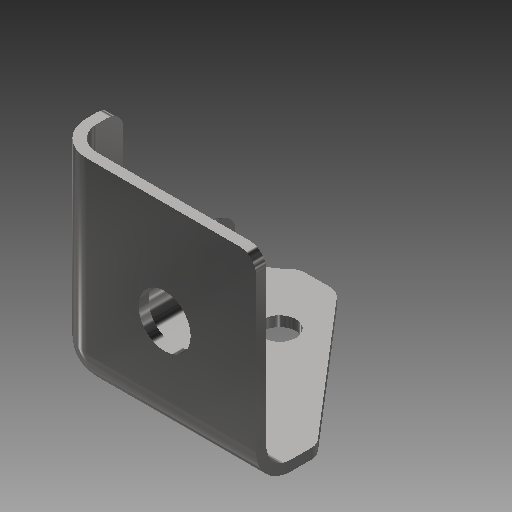
# Autodesk Inventor part: 314-06
Saved by Autodesk Inventor 2019 (Build 230136000, 136)
## iProperties
Company: Autodesk Inc.
Created: 2007-10-25
Part Number: 314-06
Document SubType Name: Modeling
Designer: Autodesk Inc.
Density: 7.85 g/cm^3
Mass: 90.2439 g
Surface Area: 99.9897 cm^2
Volume: 11.496 cm^3
Material: Steel
Description: CORNER BRACKET - L
Appearance: Steel - Polished
Component Category: Lower Component
Author: Inventor
Autodesk Inventor part; units mm, degrees
ref_plane "YZ Plane" through (0, 0, 0) normal (1, 0, 0) x (0, 1, 0)
ref_plane "XZ Plane" through (0, 0, 0) normal (0, 1, 0) x (-1, 0, 0)
ref_plane "XY Plane" through (0, 0, 0) normal (0, 0, 1) x (1, 0, 0)
sketch "Sketch1" plane through (0, 0, 0) normal (0, 0, 1) x (1, 0, 0)
  line L0 (-25, 25) -> (25, 25)
  line L1 (25, 25) -> (25, -25)
  line L2 (25, -25) -> (-25, -25)
  line L3 (-25, -25) -> (-25, 25)
  point P0 (0, 0)
  dimension "d0" = 50
  dimension "d1" = 50
  dimension "d2" = 25
  dimension "d3" = 25
  constraints: 8 end point, 2 parallel, 1 horizontal, 1 perpendicular
  measures "d0" distance of L2.end L0.start
  measures "d1" distance of L0.start L0.end
  measures "d2" distance from line of point (0, 0) L3
  measures "d3" distance from line of point (0, 0) L0
extrude "Extrusion1" add sketch "Sketch1" against normal blind 50
fillet "Fillet1" radius 8.5 3 edges at (0, -25, 0) (-25, 0, 0) (-25, -25, -25)
shell "Shell1" thickness 2.5 removed faces 3 at (-8.3333, 11.1667, -50) at (-8.3333, 25, -36.1667) at (25, 11.1667, -16.6667)
sketch "Sketch2" plane through (-25, -16.5, -8.5) normal (-1, 0, 0) x (0, 0, 1)
  line L0 (0, 41.5) -> (-41.5, 41.5) projected
  line L1 (-41.5, 41.5) -> (-41.5, 0) projected
  line L2 (-41.5, 6.5) -> (-6.5, 6.5)
  line L3 (-6.5, 6.5) -> (-6.5, 41.5)
  line L4 (-6.5, 41.5) -> (-41.5, 41.5)
  line L5 (-41.5, 41.5) -> (-41.5, 6.5)
  point P0 (8.5, 16.5)
  dimension "d8" = 35
  dimension "d9" = 35
  constraints: 8 end point, 2 parallel, 2 point on line, 1 horizontal, 1 perpendicular
  measures "d8" distance of L2.start L2.end
  measures "d9" distance from line of L2 L0.start
extrude "Extrusion2" cut sketch "Sketch2" against normal through all
sketch "Sketch3" plane through (-16.5, 25, 0) normal (0, 1, 0) x (1, 0, 0)
  line L0 (41.5, 0) -> (41.5, 2.5) projected
  line L1 (41.5, 15) -> (11.5, 50)
  line L2 (0, 50) -> (41.5, 50) projected
  line L3 (41.5, 50) -> (11.5, 50)
  line L4 (41.5, 50) -> (41.5, 15)
  point P0 (41.5, 33)
  point P1 (41.5, 8.5)
  point P2 (16.5, 0)
  point P3 (33, 50)
  point P4 (39, 50)
  dimension "d36" = 30
  dimension "d37" = 35
  constraints: 7 end point, 2 collinear, 2 point on line
  measures "d36" distance of L2.end L1.end
  measures "d37" distance of L2.end L1.start
extrude "Extrusion3" cut sketch "Sketch3" against normal through all
sketch "Sketch4" plane through (0, 0, 0) normal (0, 0, 1) x (1, 0, 0)
  line L0 (-5, -25) -> (25, -25) projected
  line L1 (-16.5, -25) -> (25, -25) projected
  line L2 (-16.5, -25) -> (-5, -25) projected
  line L3 (-25, 25) -> (-25, -10) projected
  line L4 (-25, 25) -> (-25, -16.5) projected
  line L5 (-25, -10) -> (-25, -16.5) projected
  point P0 (0, 0)
  point P1 (2.606, 0)
  dimension "d17" = 27.606
  dimension "d18" = 25
  measures "d17" distance from line of point (2.606, 0) L4
  measures "d18" distance from line of L1 point (2.606, 0)
hole "Hole1" at (2.606, 0, 0) direction (0, 0, -1) diameter 12.8 end through all
sketch "Sketch5" plane through (-16.5, -25, -8.5) normal (0, -1, 0) x (1, 0, 0)
  line L0 (12.706, 8.5) -> (25.506, 8.5) projected
  line L1 (0, 8.5) -> (41.5, 8.5) projected
  line L2 (41.5, 8.5) -> (0, 8.5) projected
  line L3 (-8.5, -6.5) -> (-8.5, -41.5) projected
  point P0 (16.5, 8.5)
  point P1 (12.285, -26.5)
  dimension "d43" = 20.785
  dimension "d44" = 35
  measures "d43" distance from line of point (12.285, -26.5) L3
  measures "d44" distance from line of point (12.285, -26.5) L0
hole "Hole2" at (-4.215, -25, -35) direction (0, 1, 0) diameter 8 end through all
sketch "Sketch6" plane through (-16.5, 25, 0) normal (0, 1, 0) x (1, 0, 0)
  arc A0 (-8.5, 8.5) -> (0, 0) centre (0, 8.5) ccw projected
  line L0 (0, 50) -> (11.5, 50) projected
  line L1 (-8.5, 15) -> (-8.5, 50) projected
  line L2 (2, 50) -> (-8.5, 40)
  line L3 (-8.5, 40) -> (-8.5, 50)
  line L4 (-8.5, 50) -> (2, 50)
  point P0 (16.5, 0)
  point P1 (9.6603, 50)
  point P2 (-8.5, 19)
  point P3 (-8.5, 46)
  dimension "d38" = 2
  dimension "d39" = 40
  constraints: 6 end point, 3 point on line, 1 collinear, 1 perpendicular
  measures "d38" horizontal distance of L2.start A0.centre
  measures "d39" vertical distance of L2.end A0.end
extrude "Extrusion4" cut sketch "Sketch6" against normal through all
fillet "Fillet3" radius 4 7 edges at (-23.75, 25, -15) (-23.75, -10, -41.1905) (-14.5, -23.75, -50) (-5, -23.75, -50) (25, -23.75, -15) (25, 25, -1.25) (-23.75, -10, -15)
equation "\"d0\" = d1"
equation "\"d2\" = 0.5 * d1"
equation "\"d3\" = 0.5 * d0"
body "Solid1"
